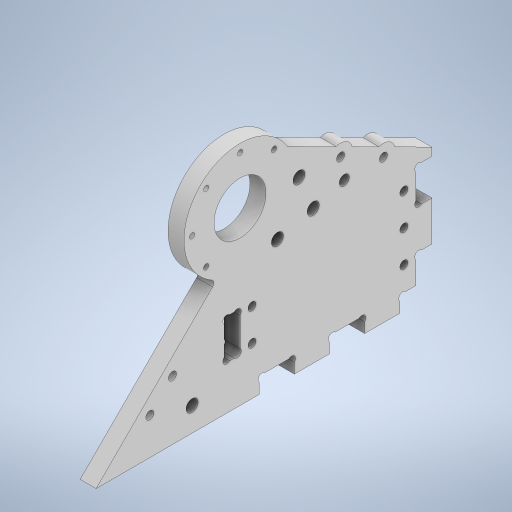
# Autodesk Inventor part: Weapon Support Wall_left
Saved by Autodesk Inventor 2023 (Build 270158000, 158)
## iProperties
Created: 2022-12-26
Part Number: Weapon Support Wall_left
Material: Generic
Document SubType Name: Modeling
Designer: justi
Density: 1 g/cm^3
Appearance: Default
Mass: 330.296 g
Surface Area: 697.211 cm^2
Volume: 330.296 cm^3
Author: justi
Autodesk Inventor part; units mm, degrees
ref_plane "YZ Plane" through (0, 0, 0) normal (1, 0, 0) x (0, 1, 0)
ref_plane "XZ Plane" through (0, 0, 0) normal (0, 1, 0) x (-1, 0, 0)
ref_plane "XY Plane" through (0, 0, 0) normal (0, 0, 1) x (1, 0, 0)
sketch "Sketch1" plane through (0, 0, 0) normal (1, 0, 0) x (0, 1, 0)
  line L0 (0, 0) -> (101.6, 0)
  line L1 (101.6, 0) -> (101.6, -165.1)
  line L2 (101.6, -165.1) -> (0, -165.1)
  line L3 (0, -165.1) -> (0, 0)
  line L4 (0, 0) -> (0, 101.6)
  line L5 (0, 101.6) -> (101.6, 0)
  circle A0 centre (135.89, -12.7) radius 38.1
  line L6 (101.6, -165.1) -> (169.8983, -29.8769)
  circle A1 centre (135.89, -12.7) radius 9.525
  point P0 (100.4115, 1.1885)
  dimension "d3" = 76.2
  dimension "d0" = 165.1
  dimension "d1" = 101.6
  dimension "d2" = 101.6
  dimension "d4" = 135.89
  dimension "d5" = 152.4
  dimension "d6" = 19.05
  constraints: 14 end point, 2 parallel, 1 centre point, 1 coincident, 1 horizontal, 1 perpendicular, 1 vertical, 4 other
  measures "d0" distance of L2.end L0.start
  measures "d1" distance of L1.end L2.end
  measures "d2" distance of L0.start L4.end
  measures "d4" distance from line of L4 point (135.89, -12.7)
  measures "d5" distance from line of L2 point (135.89, -12.7)
  measures "d6" diameter of A1
extrude "Extrusion1" add sketch "Sketch1" along normal blind 12.7
sketch "Sketch3" plane through (0, 0, 0) normal (-1, 0, 0) x (0, 0, 1)
  line L0 (-165.1, 0) -> (-165.1, 101.6) projected
  line L1 (-165.1, 95.25) -> (-152.4, 95.25)
  line L2 (-152.4, 95.25) -> (-152.4, 66.675)
  line L3 (-152.4, 66.675) -> (-165.1, 66.675)
  line L4 (-165.1, 66.675) -> (-165.1, 95.25)
  line L5 (-165.1, 34.925) -> (-152.4, 34.925)
  line L6 (-152.4, 34.925) -> (-152.4, 0)
  line L7 (-152.4, 0) -> (-165.1, 0)
  line L8 (-165.1, 0) -> (-165.1, 34.925)
  line L9 (-152.4, 0) -> (-139.7, 0)
  line L10 (-139.7, 0) -> (-139.7, 12.7)
  line L11 (-139.7, 12.7) -> (-152.4, 12.7)
  line L12 (-152.4, 12.7) -> (-152.4, 0)
  line L13 (-111.76, 0) -> (-83.82, 0)
  line L14 (-83.82, 0) -> (-83.82, 12.7)
  line L15 (-83.82, 12.7) -> (-111.76, 12.7)
  line L16 (-111.76, 12.7) -> (-111.76, 0)
  line L17 (-55.88, 0) -> (-27.94, 0)
  line L18 (-27.94, 0) -> (-27.94, 12.7)
  line L19 (-27.94, 12.7) -> (-55.88, 12.7)
  line L20 (-55.88, 12.7) -> (-55.88, 0)
  line L21 (0, 34.925) -> (-12.7, 34.925)
  line L22 (-12.7, 34.925) -> (-12.7, 66.675)
  line L23 (-12.7, 66.675) -> (0, 66.675)
  line L24 (0, 66.675) -> (0, 34.925)
  line L25 (101.6, 0) -> (-165.1, 0) projected
  point P0 (0, 0)
  point P1 (-152.4, 12.7)
  dimension "d9" = 12.7
  dimension "d10" = 28.575
  dimension "d11" = 6.35
  dimension "d12" = 12.7
  dimension "d13" = 34.925
  dimension "d14" = 31.75
  dimension "d15" = 12.7
  dimension "d16" = 12.7
  dimension "d17" = 27.94
  dimension "d18" = 12.7
  dimension "d19" = 27.94
  dimension "d20" = 12.7
  dimension "d21" = 27.94
  dimension "d22" = 27.94
  dimension "d23" = 12.7
  dimension "d24" = 31.75
  dimension "d25" = 34.925
  constraints: 48 end point, 12 parallel, 6 horizontal, 6 perpendicular, 2 point on line, 1 other
  measures "d9" distance of L2.end L3.end
  measures "d10" distance of L1.end L2.end
  measures "d11" distance from line of L1 L0.end
  measures "d12" distance of L6.end L7.end
  measures "d13" distance of L5.end L6.end
  measures "d14" distance between parallel lines of L3 L5
  measures "d15" distance of L11.end L10.end
  measures "d16" distance of L9.end L10.end
  measures "d17" distance of L15.end L14.end
  measures "d18" distance of L13.end L14.end
  measures "d19" distance of L19.end L18.end
  measures "d20" distance of L19.end L17.start
  measures "d21" distance between parallel lines of L10 L16
  measures "d22" distance between parallel lines of L20 L14
  measures "d23" distance of L22.end L23.end
  measures "d24" distance of L21.end L22.end
  measures "d25" distance of the line from the sketch origin of L21
extrude "Extrusion2" cut sketch "Sketch3" against normal blind 12.7
fillet "Fillet1" radius 3.175 1 edges at (6.35, 100.4115, 1.1885)
sketch "Sketch4" plane through (0, 0, 0) normal (-1, 0, 0) x (0, 0, 1)
  circle A0 centre (-59.5478, 133.5702) radius 5.1594
  circle A1 centre (-12.7, 135.89) radius 9.525 projected
  line L0 (-12.7, 135.89) -> (-29.8769, 169.8983)
  line L1 (-165.1, 101.6) -> (-29.8769, 169.8983) projected
  line L2 (-12.7, 135.89) -> (-80.7166, 101.5363)
  circle A2 centre (-42.3709, 99.5619) radius 5.1594
  line L3 (-59.5478, 133.5702) -> (-79.386, 123.5503)
  line L4 (-79.386, 123.5503) -> (-70.7975, 106.5462)
  circle A3 centre (-70.7975, 106.5462) radius 5.1594
  point P0 (0, 0)
  dimension "d29" = 10.3187
  dimension "d30" = 90
  dimension "d31" = 76.2
  dimension "d32" = 90
  dimension "d33" = 42.8625
  dimension "d34" = 10.3187
  dimension "d35" = 42.8625
  dimension "d36" = 19.05
  dimension "d37" = 19.05
  dimension "d39" = 22.225
  dimension "d40" = 10.3187
  constraints: 8 end point, 3 centre point, 2 point on line, 1 coincident, 1 perpendicular
  measures "d29" diameter of A0
  measures "d30" angle of L1 L0
  measures "d31" distance of L0.start L2.end
  measures "d32" angle of L0 L2
  measures "d33" distance from line of L0 L3.start
  measures "d34" diameter of A2
  measures "d35" distance from line of L0 A2.centre
  measures "d36" distance from line of L2 L3.start
  measures "d37" distance from line of L2 A2.centre
  measures "d39" distance of L3.start L3.end
  measures "d40" diameter of A3
extrude "Extrusion3" cut sketch "Sketch4" against normal blind 12.7 contours A0 | A3 L2 | L2 L4 A3 | L2 A3 L4 | A2
sketch "Sketch8" plane through (12.7, 0, 0) normal (1, 0, 0) x (0, 0, -1)
  line L0 (165.1, 101.6) -> (29.8769, 169.8983) projected
  line L1 (49.6887, 159.8918) -> (152.1117, 108.1601)
  line L2 (152.1117, 108.1601) -> (149.2489, 102.4921)
  line L3 (149.2489, 102.4921) -> (46.8259, 154.2237)
  line L4 (46.8259, 154.2237) -> (49.6887, 159.8918)
  circle A0 centre (92.5684, 131.1202) radius 9.525
  circle A1 centre (126.5767, 113.9433) radius 9.525
  point P0 (0, 0)
  point P1 (123.1024, 122.8121)
  point P2 (135.7766, 116.4106)
  point P3 (89.0941, 139.9889)
  point P4 (101.7683, 133.5875)
  dimension "d51" = 6.35
  dimension "d52" = 19.05
  dimension "d53" = 19.05
  dimension "d54" = 38.1
  dimension "d61" = 25.4
  constraints: 8 end point, 4 point on line, 2 centre point, 2 parallel, 1 perpendicular
  measures "d51" distance of L1.end L2.end
  measures "d52" diameter of A0
  measures "d53" diameter of A1
  measures "d54" distance of A1.centre A0.centre
  measures "d61" distance from line of L2 A1.centre
extrude "Extrusion6" add sketch "Sketch8" against normal blind 12.7 contours L0 A1 | L0 A0
sketch "Sketch9" plane through (12.7, 0, 0) normal (1, 0, 0) x (0, 0, -1)
  arc A0 (101.7683, 133.5875) -> (89.0941, 139.9889) centre (92.5684, 131.1202) ccw projected
  circle A1 centre (92.5684, 131.1202) radius 3.175
  arc A2 (135.7766, 116.4106) -> (123.1024, 122.8121) centre (126.5767, 113.9433) ccw projected
  circle A3 centre (126.5767, 113.9433) radius 3.175
  point P0 (0, 0)
  dimension "d57" = 6.35
  dimension "d58" = 6.35
  constraints: 2 centre point, 2 coincident
  measures "d57" diameter of A1
  measures "d58" diameter of A3
extrude "Extrusion7" cut sketch "Sketch9" against normal blind 12.7
sketch "Sketch11" plane through (12.7, 0, 0) normal (1, 0, 0) x (0, 0, -1)
  circle A0 centre (12.7, 135.89) radius 9.525 projected
  circle A1 centre (12.7, 135.89) radius 20.6375
  point P0 (0, 0)
  dimension "d62" = 41.275
  constraints: 1 centre point, 1 coincident
  measures "d62" diameter of A1
extrude "Extrusion8" cut sketch "Sketch11" against normal blind 25.4
sketch "Sketch12" plane through (12.7, 0, 0) normal (1, 0, 0) x (0, 0, -1)
  line L0 (152.4, 95.25) -> (152.4, 66.675) projected
  line L1 (152.4, 95.25) -> (154.6451, 93.0049)
  line L2 (152.4, 95.25) -> (165.1, 95.25) projected
  line L3 (152.4, 66.675) -> (165.1, 66.675) projected
  line L4 (152.4, 66.675) -> (154.6451, 68.9201)
  line L5 (152.4, 34.925) -> (152.4, 12.7) projected
  line L6 (152.4, 34.925) -> (154.6451, 32.6799)
  line L7 (152.4, 34.925) -> (165.1, 34.925) projected
  line L8 (139.7, 12.7) -> (139.7, 0) projected
  line L9 (139.7, 12.7) -> (141.9451, 10.4549)
  line L10 (139.7, 12.7) -> (152.4, 12.7) projected
  line L11 (83.82, 12.7) -> (83.82, 0) projected
  line L12 (83.82, 12.7) -> (86.0651, 10.4549)
  line L13 (83.82, 12.7) -> (111.76, 12.7) projected
  line L14 (111.76, 0) -> (111.76, 12.7) projected
  line L15 (111.76, 12.7) -> (109.5149, 10.4549)
  line L16 (27.94, 12.7) -> (27.94, 0) projected
  line L17 (27.94, 12.7) -> (30.1851, 10.4549)
  line L18 (27.94, 12.7) -> (55.88, 12.7) projected
  line L19 (55.88, 0) -> (55.88, 12.7) projected
  line L20 (55.88, 12.7) -> (53.6349, 10.4549)
  circle A0 centre (154.6451, 93.0049) radius 3.175
  circle A1 centre (154.6451, 68.9201) radius 3.175
  circle A2 centre (154.6451, 32.6799) radius 3.175
  circle A3 centre (141.9451, 10.4549) radius 3.175
  circle A4 centre (109.5149, 10.4549) radius 3.175
  circle A5 centre (86.0651, 10.4549) radius 3.175
  circle A6 centre (53.6349, 10.4549) radius 3.175
  circle A7 centre (30.1851, 10.4549) radius 3.175
  line L21 (12.7, 66.675) -> (0, 66.675) projected
  line L22 (0, 66.675) -> (2.2451, 64.4299)
  line L23 (12.7, 66.675) -> (10.4549, 64.4299)
  line L24 (12.7, 66.675) -> (12.7, 34.925) projected
  line L25 (0, 34.925) -> (12.7, 34.925) projected
  line L26 (0, 34.925) -> (2.2451, 37.1701)
  line L27 (12.7, 34.925) -> (10.4549, 37.1701)
  circle A8 centre (2.2451, 64.4299) radius 3.175
  circle A9 centre (10.4549, 64.4299) radius 3.175
  circle A10 centre (2.2451, 37.1701) radius 3.175
  circle A11 centre (10.4549, 37.1701) radius 3.175
  point P0 (0, 0)
  dimension "d65" = 3.175
  dimension "d66" = 45
  dimension "d67" = 3.175
  dimension "d68" = 45
  dimension "d69" = 3.175
  dimension "d70" = 45
  dimension "d71" = 3.175
  dimension "d72" = 45
  dimension "d73" = 3.175
  dimension "d74" = 45
  dimension "d75" = 3.175
  dimension "d76" = 45
  dimension "d77" = 3.175
  dimension "d78" = 45
  dimension "d79" = 3.175
  dimension "d80" = 45
  dimension "d81" = 6.35
  dimension "d82" = 6.35
  dimension "d83" = 6.35
  dimension "d84" = 6.35
  dimension "d85" = 6.35
  dimension "d86" = 6.35
  dimension "d87" = 6.35
  dimension "d88" = 6.35
  dimension "d89" = 3.175
  dimension "d90" = 45
  dimension "d91" = 3.175
  dimension "d92" = 45
  dimension "d93" = 3.175
  dimension "d94" = 45
  dimension "d95" = 3.175
  dimension "d96" = 45
  dimension "d97" = 6.35
  dimension "d98" = 6.35
  dimension "d99" = 6.35
  dimension "d100" = 6.35
  constraints: 24 end point, 12 centre point, 10 point on line
  measures "d65" distance of L0.start L1.end
  measures "d66" angle of L2 L1
  measures "d67" distance of L0.end L4.end
  measures "d68" angle of L3 L4
  measures "d69" distance of L5.start L6.end
  measures "d70" angle of L7 L6
  measures "d71" distance of L8.start L9.end
  measures "d72" angle of L10 L9
  measures "d73" distance of L11.start L12.end
  measures "d74" angle of L13 L12
  measures "d75" distance of L13.end L15.end
  measures "d76" angle of L14 L15
  measures "d77" distance of L16.start L17.end
  measures "d78" angle of L18 L17
  measures "d79" distance of L18.end L20.end
  measures "d80" angle of L19 L20
  measures "d81" diameter of A0
  measures "d82" diameter of A1
  measures "d83" diameter of A2
  measures "d84" diameter of A3
  measures "d85" diameter of A4
  measures "d86" diameter of A5
  measures "d87" diameter of A6
  measures "d88" diameter of A7
  measures "d89" distance of L21.end L22.end
  measures "d90" angle of L21 L22
  measures "d91" distance of L21.start L23.end
  measures "d92" angle of L24 L23
  measures "d93" distance of L25.start L26.end
  measures "d94" angle of L25 L26
  measures "d95" distance of L24.end L27.end
  measures "d96" angle of L24 L27
  measures "d97" diameter of A8
  measures "d98" diameter of A9
  measures "d99" diameter of A10
  measures "d100" diameter of A11
extrude "Extrusion9" cut sketch "Sketch12" against normal blind 12.7
sketch "Sketch14" plane through (12.7, 0, 0) normal (1, 0, 0) x (0, 0, -1)
  line L0 (152.4, 12.7) -> (152.4, 30.4349) projected
  line L1 (144.1901, 12.7) -> (152.4, 12.7) projected
  line L2 (152.4, 71.1651) -> (152.4, 90.7599) projected
  circle A0 centre (142.875, 69.85) radius 3.175
  circle A1 centre (142.875, 44.45) radius 3.175
  line L3 (-4.4104, 97.1896) -> (-101.6, 0) projected
  circle A2 centre (-58.9438, 29.1858) radius 3.175
  circle A3 centre (-40.9833, 47.1463) radius 3.175
  circle A4 centre (22.225, 44.45) radius 3.175
  circle A5 centre (22.225, 69.85) radius 3.175
  line L4 (32.4301, 12.7) -> (51.3899, 12.7) projected
  line L5 (12.7, 62.1849) -> (12.7, 39.4151) projected
  point P0 (0, 0)
  dimension "d112" = 6.35
  dimension "d114" = 9.525
  dimension "d115" = 6.35
  dimension "d116" = 9.525
  dimension "d121" = 6.35
  dimension "d123" = 6.35
  dimension "d127" = 6.35
  dimension "d128" = 6.35
  dimension "d129" = 31.75
  dimension "d130" = 25.4
  dimension "d131" = 9.525
  dimension "d132" = 9.525
  constraints: 6 centre point
  measures "d112" diameter of A0
  measures "d114" distance from line of L2 A0.centre
  measures "d115" diameter of A1
  measures "d116" distance from line of L2 A1.centre
  measures "d121" diameter of A2
  measures "d123" diameter of A3
  measures "d127" diameter of A4
  measures "d128" diameter of A5
  measures "d129" distance from line of L4 A4.centre
  measures "d130" distance of A4.centre A5.centre
  measures "d131" distance from line of L5 A4.centre
  measures "d132" distance from line of L5 A5.centre
extrude "Extrusion10" cut sketch "Sketch14" against normal blind 12.7
sketch "Sketch16" plane through (12.7, 0, 0) normal (1, 0, 0) x (0, 0, -1)
  circle A0 centre (142.875, 57.15) radius 3.175
  circle A1 centre (142.875, 69.85) radius 3.175 projected
  circle A2 centre (142.875, 82.55) radius 3.175
  line L0 (152.4, 71.1651) -> (152.4, 90.7599) projected
  circle A3 centre (142.875, 31.75) radius 3.175
  line L1 (152.4, 12.7) -> (152.4, 30.4349) projected
  circle A4 centre (142.875, 44.45) radius 3.175 projected
  line L2 (144.1901, 12.7) -> (152.4, 12.7) projected
  point P0 (0, 0)
  dimension "d152" = 6.35
  dimension "d154" = 6.35
  dimension "d156" = 9.525
  dimension "d157" = 9.525
  dimension "d158" = 6.35
  dimension "d159" = 9.525
  dimension "d161" = 19.05
  dimension "d162" = 25.4
  dimension "d163" = 25.4
  constraints: 3 centre point
  measures "d152" diameter of A0
  measures "d154" diameter of A2
  measures "d156" distance from line of L0 A2.centre
  measures "d157" distance from line of L0 A0.centre
  measures "d158" diameter of A3
  measures "d159" distance from line of L1 A3.centre
  measures "d161" distance from line of L2 A3.centre
  measures "d162" distance of A3.centre A0.centre
  measures "d163" distance of A2.centre A0.centre
extrude "Extrusion12" cut sketch "Sketch16" against normal blind 12.7 contours A0 | A2 | A3
sketch "Sketch17" plane through (12.7, 0, 0) normal (1, 0, 0) x (0, 0, -1)
  circle A0 centre (142.875, 69.85) radius 3.175 projected
  circle A1 centre (142.875, 69.85) radius 3.175
  circle A2 centre (142.875, 44.45) radius 3.175 projected
  circle A3 centre (142.875, 44.45) radius 3.175
  point P0 (0, 0)
  dimension "d166" = 6.35
  dimension "d167" = 6.35
  constraints: 2 centre point, 2 coincident
  measures "d166" diameter of A1
  measures "d167" diameter of A3
extrude "Extrusion13" add sketch "Sketch17" against normal blind 12.7
sketch "Sketch18" plane through (12.7, 0, 0) normal (1, 0, 0) x (0, 0, -1)
  circle A0 centre (22.225, 63.5) radius 3.175
  circle A1 centre (22.225, 38.1) radius 3.175
  line L0 (12.7, 62.1849) -> (12.7, 39.4151) projected
  circle A2 centre (22.225, 69.85) radius 3.175 projected
  point P0 (0, 0)
  dimension "d170" = 6.35
  dimension "d171" = 6.35
  dimension "d172" = 9.525
  dimension "d173" = 9.525
  dimension "d174" = 25.4
  dimension "d175" = 6.35
  constraints: 2 centre point
  measures "d170" diameter of A0
  measures "d171" diameter of A1
  measures "d172" distance from line of L0 A0.centre
  measures "d173" distance from line of L0 A1.centre
  measures "d174" distance of A0.centre A1.centre
  measures "d175" distance of A2.centre A0.centre
extrude "Extrusion14" cut sketch "Sketch18" against normal blind 12.7 contours A0 | A1
sketch "Sketch19" plane through (12.7, 0, 0) normal (1, 0, 0) x (0, 0, -1)
  circle A0 centre (22.225, 69.85) radius 3.175 projected
  circle A1 centre (22.225, 69.85) radius 3.175
  circle A2 centre (22.225, 44.45) radius 3.175 projected
  circle A3 centre (22.225, 44.45) radius 3.175
  point P0 (0, 0)
  point P1 (22.225, 66.675)
  point P2 (22.225, 41.275)
  dimension "d178" = 6.35
  dimension "d179" = 6.35
  constraints: 2 centre point, 2 coincident, 2 vertical alignment
  measures "d178" diameter of A1
  measures "d179" diameter of A3
extrude "Extrusion15" add sketch "Sketch19" against normal blind 12.7
sketch "Sketch21" plane through (12.7, 0, 0) normal (1, 0, 0) x (0, 0, -1)
  circle A0 centre (12.7, 135.89) radius 20.6375 projected
  line L0 (12.7, 135.89) -> (151.9072, 135.89)
  line L1 (12.7, 135.89) -> (95.504, 113.7027)
  line L2 (65.5985, 121.7159) -> (12.7, 135.89)
  circle A1 centre (95.504, 113.7027) radius 3.9688
  point P0 (0, 0)
  dimension "d182" = 15
  dimension "d184" = 85.725
  dimension "d185" = 7.9375
  constraints: 6 end point, 2 point on line, 1 centre point, 1 coincident, 1 horizontal
  measures "d182" angle of L1 L0
  measures "d184" distance of L0.start L1.end
  measures "d185" diameter of A1
extrude "Extrusion16" cut sketch "Sketch21" against normal blind 12.7 contours A1
sketch "Sketch24" plane through (12.7, 0, 0) normal (1, 0, 0) x (0, 0, -1)
  circle A0 centre (12.7, 135.89) radius 20.6375 projected
  circle A1 centre (12.7, 135.89) radius 44.45
  circle A2 centre (59.5478, 133.5702) radius 5.1594 projected
  circle A3 centre (59.5478, 133.5702) radius 5.1594
  circle A4 centre (42.3709, 99.5619) radius 5.1594 projected
  circle A5 centre (42.3709, 99.5619) radius 5.1594
  circle A6 centre (12.7, 135.89) radius 20.6375
  point P0 (0, 0)
  point P1 (37.2619, 98.8425)
  point P2 (44.096, 104.4243)
  point P3 (56.6582, 129.2959)
  point P4 (57.0946, 138.109)
  dimension "d193" = 88.9
  constraints: 4 centre point, 4 coincident, 1 concentric
  measures "d193" diameter of A1
extrude "Extrusion19" add sketch "Sketch24" against normal blind 12.7 contours A2 A1 A4
fillet "Fillet2" radius 3.175 1 edges at (6.35, 95.576, 6.024)
sketch "Sketch30" plane through (12.7, 0, 0) normal (1, 0, 0) x (0, 0, -1)
  circle A0 centre (-25.4, 19.05) radius 4.7625
  point P0 (0, 0)
  dimension "d209" = 9.525
  dimension "d210" = 25.4
  dimension "d211" = 19.05
  constraints: 1 centre point
  measures "d209" diameter of A0
  measures "d210" horizontal distance of point (0, 0) A0.centre
  measures "d211" vertical distance of A0.centre point (0, 0)
extrude "Extrusion22" cut sketch "Sketch30" against normal blind 12.7
sketch "Sketch32" plane through (12.7, 0, 0) normal (1, 0, 0) x (0, 0, -1)
  circle A0 centre (59.5478, 133.5702) radius 5.1594 projected
  circle A1 centre (59.5478, 133.5702) radius 4.7625
  circle A2 centre (70.7975, 106.5462) radius 5.1594 projected
  circle A3 centre (70.7975, 106.5462) radius 4.7625
  circle A4 centre (42.3709, 99.5619) radius 5.1594 projected
  circle A5 centre (42.3709, 99.5619) radius 4.7625
  circle A6 centre (59.5478, 133.5702) radius 5.1594
  circle A7 centre (70.7975, 106.5462) radius 5.1594
  circle A8 centre (42.3709, 99.5619) radius 5.1594
  point P0 (0, 0)
  dimension "d227" = 9.525
  dimension "d228" = 9.525
  dimension "d229" = 9.525
  constraints: 6 centre point, 6 coincident, 3 concentric
  measures "d227" diameter of A1
  measures "d228" diameter of A3
  measures "d229" diameter of A5
extrude "Extrusion24" add sketch "Sketch32" against normal blind 12.7
sketch "Sketch33" plane through (12.7, 0, 0) normal (1, 0, 0) x (0, 0, -1)
  circle A0 centre (12.7, 135.89) radius 20.6375 projected
  circle A1 centre (12.7, 135.89) radius 31.75
  line L0 (12.7, 135.89) -> (12.7, 173.99)
  line L1 (12.7, 135.89) -> (-14.2408, 162.8308)
  line L2 (12.7, 135.89) -> (39.6408, 162.8308)
  line L3 (12.7, 135.89) -> (-25.4, 135.89)
  line L4 (12.7, 135.89) -> (-14.2408, 108.9492)
  circle A2 centre (12.7, 173.99) radius 2.0828
  circle A3 centre (39.6408, 162.8308) radius 2.0828
  circle A4 centre (-14.2408, 162.8308) radius 2.0828
  circle A5 centre (-25.4, 135.89) radius 2.0828
  circle A6 centre (-14.2408, 108.9492) radius 2.0828
  point P0 (0, 0)
  dimension "d232" = 63.5
  dimension "d233" = 38.1
  dimension "d234" = 38.1
  dimension "d235" = 45
  dimension "d236" = 38.1
  dimension "d237" = 45
  dimension "d238" = 38.1
  dimension "d239" = 38.1
  dimension "d240" = 45
  dimension "d241" = 4.1656
  dimension "d242" = 4.1656
  dimension "d243" = 4.1656
  dimension "d244" = 4.1656
  dimension "d245" = 4.1656
  constraints: 10 end point, 6 centre point, 4 coincident, 2 point on line, 1 horizontal, 1 vertical
  measures "d232" diameter of A1
  measures "d233" distance of L0.start L0.end
  measures "d234" distance of L0.start L1.end
  measures "d235" angle of L0 L1
  measures "d236" distance of L0.start L2.end
  measures "d237" angle of L0 L2
  measures "d238" distance of L0.start L3.end
  measures "d239" distance of L0.start L4.end
  measures "d240" angle of L3 L4
  measures "d241" diameter of A2
  measures "d242" diameter of A3
  measures "d243" diameter of A4
  measures "d244" diameter of A5
  measures "d245" diameter of A6
extrude "Extrusion25" cut sketch "Sketch33" against normal blind 12.7 contours A2 | A3 | A4 | A5 | A6
body "Solid1"
